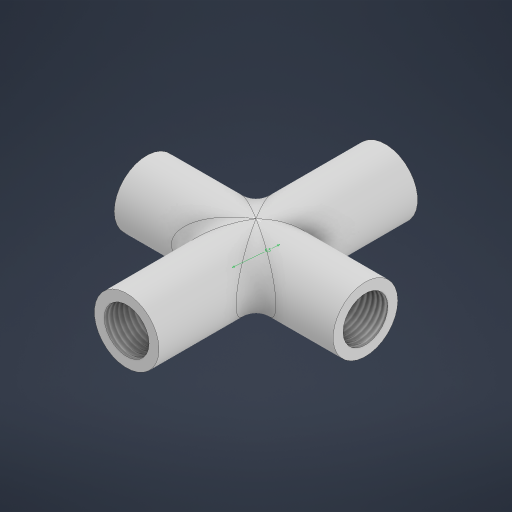
# Autodesk Inventor part: Part2
Saved by Autodesk Inventor 2023 (Build 270158030, 158C)
## iProperties
Created: 2023-02-03
Part Number: Part2
Material: Generic
Document SubType Name: Modeling
Designer: Monster
Density: 1 g/cm^3
Appearance: Default
Author: Monster
Autodesk Inventor part; units mm, degrees
ref_plane "YZ Plane" through (0, 0, 0) normal (1, 0, 0) x (0, 1, 0)
ref_plane "XZ Plane" through (0, 0, 0) normal (0, 1, 0) x (-1, 0, 0)
ref_plane "XY Plane" through (0, 0, 0) normal (0, 0, 1) x (1, 0, 0)
sketch "Sketch1" plane through (0, 0, 0) normal (0, 0, 1) x (1, 0, 0)
  circle A0 centre (0, 0) radius 3.25
  dimension "d0" = 6.5
  constraints: 1 centre point, 1 coincident
  measures "d0" diameter of A0
extrude "Extrusion1" add sketch "Sketch1" along normal blind 13
sketch "Sketch2" plane through (0, 0, 13) normal (0, 0, 1) x (1, 0, 0)
  circle A0 centre (0, 0) radius 4.25
  dimension "d3" = 8.5
  constraints: 1 centre point, 1 coincident
  measures "d3" diameter of A0
extrude "Extrusion2" cut sketch "Sketch2" along normal blind 2
pattern_circular "Circular Pattern1" count 4 over 360 about axis through (0, -10, 0) along (0, 1, 0) of "Extrusion1", "Extrusion2"
fillet "Fillet1" radius 2 6 edges at (2.2981, -2.2981, 2.2981) (2.2981, 2.2981, 2.2981) (-2.2981, -2.2981, 2.2981) (-2.2981, 2.2981, 2.2981) (-2.2981, 2.2981, -2.2981) (-2.2981, -2.2981, -2.2981)
sketch "Sketch3" plane through (0, 0, 13) normal (0, 0, 1) x (1, 0, 0)
  circle A0 centre (0, 0) radius 2.25
  dimension "d10" = 4.5
  constraints: 1 centre point, 1 coincident
  measures "d10" diameter of A0
extrude "Extrusion3" cut sketch "Sketch3" against normal blind 6
thread "Thread1" size "M3x0.5" class "6H" standard "ANSI Metric M Profile" length 8
pattern_circular "Circular Pattern2" count 4 over 360 about axis through (0, -10, 0) along (0, 1, 0) of "Extrusion3"
thread "Thread2" size "M3x0.5" class "6H" standard "ANSI Metric M Profile" length 8
sketch "Sketch4" plane through (13, 0, 0) normal (1, 0, 0) x (0, 0, -1)
  circle A0 centre (0, 0) radius 3.25
  constraints: 1 centre point, 1 coincident
extrude "Extrusion4" cut sketch "Sketch4" against normal blind 3
sketch "Sketch5" plane through (-13, 0, 0) normal (-1, 0, 0) x (0, 0, 1)
  circle A0 centre (0, 0) radius 3.25
  constraints: 1 centre point, 1 coincident
extrude "Extrusion5" cut sketch "Sketch5" against normal blind 3
sketch "Sketch6" plane through (10, 0, 0) normal (1, 0, 0) x (0, 0, -1)
  circle A0 centre (0, 0) radius 2.25
  circle A1 centre (0, 0) radius 3.25
  constraints: 2 centre point, 2 coincident
extrude "Extrusion6" cut sketch "Sketch6" against normal blind 6 contours A0
sketch "Sketch7" plane through (-10, 0, 0) normal (-1, 0, 0) x (0, 0, 1)
  circle A0 centre (0, 0) radius 2.25
  circle A1 centre (0, 0) radius 3.25
  constraints: 2 centre point, 2 coincident
extrude "Extrusion7" cut sketch "Sketch7" against normal blind 6 contours A0
sketch "Sketch8" plane through (0, 0, 13) normal (0, 0, 1) x (1, 0, 0)
  circle A0 centre (0, 0) radius 2.25
  constraints: 1 centre point, 1 coincident
extrude "Extrusion8" cut sketch "Sketch8" against normal blind 8
sketch "Sketch9" plane through (0, 0, -13) normal (0, 0, -1) x (-1, 0, 0)
  circle A0 centre (0, 0) radius 2.25
  constraints: 1 centre point, 1 coincident
extrude "Extrusion9" cut sketch "Sketch9" against normal blind 8
extrude "Extrusion10" add sketch "Sketch6" along normal blind 1
extrude "Extrusion11" add sketch "Sketch7" along normal blind 1
thread "Thread7" size "M3x0.5" class "6H" standard "ANSI Metric M Profile" length 6
thread "Thread8" size "M3x0.5" class "6H" standard "ANSI Metric M Profile" length 6
body "Solid1"
